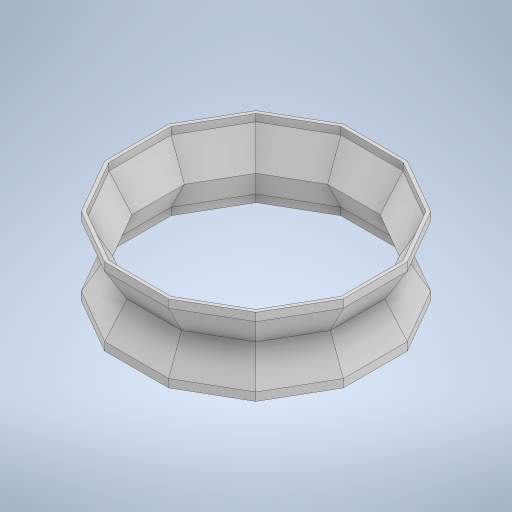
# Autodesk Inventor part: OV-PAM_n_12_standard_1F
Saved by Autodesk Inventor 2024 (Build 280153000, 153)
## iProperties
Created: 2023-08-31
Part Number: OV-PAM_n_12_standard_1F
Material: 일반
Document SubType Name: Modeling
Designer: jsw
Density: 1 g/cm^3
Appearance: 기본값
Author: jsw
Autodesk Inventor part; units mm, degrees
ref_plane "YZ Plane" through (0, 0, 0) normal (1, 0, 0) x (0, 1, 0)
sketch "스케치1" plane through (0, 0, 0) normal (0, 1, 0) x (-1, 0, 0)
  line L0 (-4.5652, 17.0375) -> (4.5652, 17.0375)
  line L1 (4.5652, 17.0375) -> (12.4723, 12.4723)
  line L2 (12.4723, 12.4723) -> (17.0375, 4.5652)
  line L3 (17.0375, 4.5652) -> (17.0375, -4.5652)
  line L4 (17.0375, -4.5652) -> (12.4723, -12.4723)
  line L5 (12.4723, -12.4723) -> (4.5652, -17.0375)
  line L6 (4.5652, -17.0375) -> (-4.5652, -17.0375)
  line L7 (-4.5652, -17.0375) -> (-12.4723, -12.4723)
  line L8 (-12.4723, -12.4723) -> (-17.0375, -4.5652)
  line L9 (-17.0375, -4.5652) -> (-17.0375, 4.5652)
  line L10 (-17.0375, 4.5652) -> (-12.4723, 12.4723)
  line L11 (-12.4723, 12.4723) -> (-4.5652, 17.0375)
  line L12 (4.7259, -17.6375) -> (-4.7259, -17.6375)
  line L13 (-4.7259, -17.6375) -> (-12.9115, -12.9115)
  line L14 (-12.9115, -12.9115) -> (-17.6375, -4.7259)
  line L15 (-17.6375, -4.7259) -> (-17.6375, 4.7259)
  line L16 (-17.6375, 4.7259) -> (-12.9115, 12.9115)
  line L17 (-12.9115, 12.9115) -> (-4.7259, 17.6375)
  line L18 (-4.7259, 17.6375) -> (4.7259, 17.6375)
  line L19 (4.7259, 17.6375) -> (12.9115, 12.9115)
  line L20 (12.9115, 12.9115) -> (17.6375, 4.7259)
  line L21 (17.6375, 4.7259) -> (17.6375, -4.7259)
  line L22 (17.6375, -4.7259) -> (12.9115, -12.9115)
  line L23 (12.9115, -12.9115) -> (4.7259, -17.6375)
  point P0 (0, 0)
  point P1 (0, 0)
  point P2 (0, 0)
  dimension "d1" = 35.277
  dimension "d2" = 0.6
  constraints: 48 end point, 2 coincident, 2 horizontal, 50 other
  measures "d1" distance of L8.end L2.end
  measures "d2" distance between parallel lines of L3 L21
extrude "돌출1" add sketch "스케치1" along normal blind 4.5 contours L0 L1 L2 L3 L4 L5 L6 L7 L8 L9 L10 L11 | L12 L13 L14 L15 L16 L17 L18 L19 L20 L21 L22 L23
ref_plane "작업 평면1" through (12.9115, 0, 12.9115) normal (-0.75, -0.5, -0.4330127) x (0.5, 0, -0.8660254)
sketch "스케치2" plane through (17.6375, 0, 4.7259) normal (0.8660254, 0, 0.5) x (0.5, 0, -0.8660254)
  line L0 (-9.4519, 0) -> (0, 0) projected
  line L1 (0, 0) -> (0, 4.5) projected
  line L2 (-9.4519, 4.5) -> (0, 4.5) projected
  line L3 (-9.4519, 0) -> (-9.4519, 4.5) projected
  line L4 (-9.4519, 0) -> (-17.6375, 0) projected
  line L5 (-9.4519, 0) -> (-17.2461, 4.5)
  line L6 (-9.4519, 4.5) -> (-17.6375, 4.5) projected
  line L7 (0, 0) -> (-0.5, 4.5)
  line L8 (-9.4519, 4.5) -> (-17.2461, 4.5)
  point P0 (-4.7259, 0)
  point P1 (-17.6375, 9)
  dimension "d6" = 150
  dimension "d7" = 0.5
  constraints: 6 end point, 2 point on line, 1 collinear
  measures "d6" angle of L5 L0
  measures "d7" distance of L1.end L7.end
extrude "돌출2" cut sketch "스케치2" along normal up to surface contours L3 L2 L7 L0 | L5 L6 L3 surface through (12.9115, 0, 12.9115) normal (-0.75, -0.5, -0.4330127)
pattern_circular "원형 패턴1" count 12 over 360 about axis through (0, -10, 0) along (0, 1, 0) of "돌출2"
sketch "스케치3" plane through (0, 0, 0) normal (0, -1, 0) x (1, 0, 0)
  line L0 (-12.9115, -12.9115) -> (-17.6375, -4.7259) projected
  line L1 (-4.7259, -17.6375) -> (-12.9115, -12.9115) projected
  line L2 (4.7259, -17.6375) -> (-4.7259, -17.6375) projected
  line L3 (12.9115, -12.9115) -> (4.7259, -17.6375) projected
  line L4 (17.6375, -4.7259) -> (12.9115, -12.9115) projected
  line L5 (17.6375, 4.7259) -> (17.6375, -4.7259) projected
  line L6 (12.9115, 12.9115) -> (17.6375, 4.7259) projected
  line L7 (4.7259, 17.6375) -> (12.9115, 12.9115) projected
  line L8 (-4.7259, 17.6375) -> (4.7259, 17.6375) projected
  line L9 (-12.9115, 12.9115) -> (-4.7259, 17.6375) projected
  line L10 (-17.6375, 4.7259) -> (-12.9115, 12.9115) projected
  line L11 (-17.6375, -4.7259) -> (-17.6375, 4.7259) projected
  point P0 (0, 0)
extrude "돌출3" add sketch "스케치3" along normal blind 1.2
ref_plane "작업 평면2" through (0, 4.5, 0) normal (0, 1, 0) x (1, 0, 0)
mirror "미러1" about plane through (0, 4.5, 0) normal (0, 1, 0) of "돌출2", "원형 패턴1", "돌출3", "돌출1"
shell "쉘1" thickness 0.5 removed faces 2 at (-1.5753, 10.2, 5.8792) at (-1.5753, -1.2, 5.8792)
